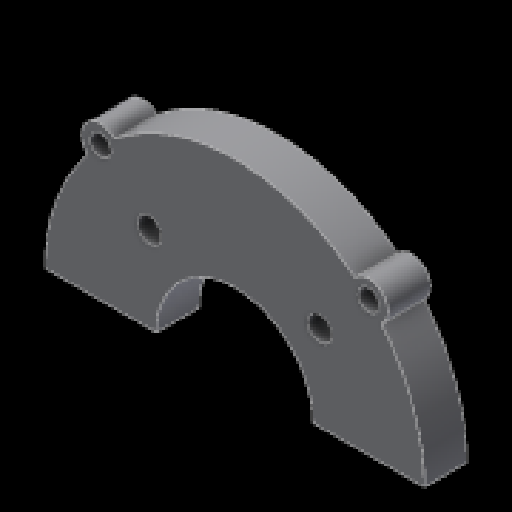
# Autodesk Inventor part: CimCoderMount
Saved by Autodesk Inventor 2025.2 (Build 292293000, 293)
## iProperties
Created: 2026-01-26
Part Number: CimCoderMount
Material: Generic
Document SubType Name: Sheet Metal
Designer: valer
Density: 1 g/cm^3
Appearance: Default
Sheet Metal Rule: Default
Author: valer
Autodesk Inventor part; units mm, degrees
ref_plane "YZ Plane" through (0, 0, 0) normal (1, 0, 0) x (0, 1, 0)
ref_plane "XZ Plane" through (0, 0, 0) normal (0, 1, 0) x (-1, 0, 0)
ref_plane "XY Plane" through (0, 0, 0) normal (0, 0, 1) x (1, 0, 0)
sketch "Base" plane through (0, 0, 0) normal (0, 0, 1) x (1, 0, 0)
  circle A0 centre (0, 0) radius 50.8
  circle A1 centre (0, 0) radius 16.5
  line L0 (-71.12, 0) -> (71.12, 0)
  line L1 (0, -71.12) -> (0, 71.12) construction
  circle A2 centre (-17.9605, 17.9605) radius 2.5527
  circle A3 centre (17.9605, 17.9605) radius 2.5527
  circle A4 centre (17.9605, -17.9605) radius 2.5527
  circle A5 centre (-17.9605, -17.9605) radius 2.5527
  circle A6 centre (0, 0) radius 16 construction
  circle A7 centre (0, 0) radius 40
  line L2 (0, 0) -> (28.2843, 28.2843) construction
  circle A8 centre (28.2843, 28.2843) radius 2.2
  circle A9 centre (-28.2843, 28.2843) radius 2.2
  circle A10 centre (28.2843, -28.2843) radius 2.2
  circle A11 centre (-28.2843, -28.2843) radius 2.2
  circle A12 centre (28.2843, 28.2843) radius 4
  circle A13 centre (17.9605, 17.9605) radius 4
  circle A14 centre (-17.9605, 17.9605) radius 4
  circle A15 centre (-28.2843, 28.2843) radius 4
  line L3 (0, 0) -> (35.921, 35.921)
  line L4 (0, 0) -> (-35.921, 35.921)
  circle A16 centre (28.2843, -28.2843) radius 4
  circle A17 centre (-28.2843, -28.2843) radius 4
  circle A18 centre (17.9605, -17.9605) radius 4
  circle A19 centre (-17.9605, -17.9605) radius 4
  point P0 (-25.4558, 25.4558)
  point P1 (-20.7889, 20.7889)
  point P2 (-15.1321, 15.1321)
  point P3 (-11.6673, 11.6673)
  point P4 (11.6673, 11.6673)
  point P5 (15.1321, 15.1321)
  point P6 (20.7889, 20.7889)
  point P7 (25.4558, 25.4558)
  point P8 (31.1127, 31.1127)
  point P9 (-31.1127, 31.1127)
  point P10 (25.318, 30.9677)
  point P11 (-25.318, 30.9677)
  point P12 (-30.9677, 25.318)
  point P13 (-40, 0)
  point P14 (-16.5, 0)
  point P15 (16.5, 0)
  point P16 (40, 0)
  point P17 (30.9677, 25.318)
  point P18 (30.9677, -25.318)
  point P19 (-30.9677, -25.318)
  point P20 (-25.318, -30.9677)
  point P21 (25.318, -30.9677)
  dimension "d26" = 80
  dimension "d0" = 101.6
  dimension "d25" = 0.5
  dimension "d27" = 4.4
  dimension "d29" = 8
  measures "d0" diameter of A0
  measures "d25" radial gap between concentric circles of A1 A6
  measures "d27" diameter of A8
  measures "d29" diameter of A12
extrude "Plate1" add sketch "Base" along normal blind 9 contours A7 A16 A17 L0 A1 | L0 A1 L3 A13 A12 A7 | L3 A8 A7 A12 | A12 A7 A8 L3 | A7 A15 L4 A14 A1 L0 | A12 L3 A8 A7 | A16 A7 A10 | A7 A10 A16 | L4 A9 A7 A15 | A15 A7 A9 L4 | A12 L3 A13 A1 L4 A14 A15 A7 | A7 A8 L3 A12 | A7 A9 L4 A15 | A17 A7 A11 | A7 A11 A17 | A15 L4 A9 A7 | L3 A3 A13 | A13 L3 A3 | L4 A2 A14 | A14 L4 A2 | A18 | A19
fillet "Fillet2" radius 6 8 edges at (-30.9677, 25.318, 4.5) (-30.9677, -25.318, 4.5) (-25.318, -30.9677, 4.5) (25.318, -30.9677, 4.5) (30.9677, -25.318, 4.5) (30.9677, 25.318, 4.5) (25.318, 30.9677, 4.5) (-25.318, 30.9677, 4.5)
equation "\"d28\" = Thickness"
equation "\"BendRadius\" = Thickness"
equation "\"BendReliefWidth\" = Thickness"
equation "\"BendReliefDepth\" = 0.5 * Thickness"
equation "\"CornerReliefSize\" = 4 * Thickness"
equation "\"MinimumRemnant\" = 2 * Thickness"
equation "\"TransitionRadius\" = BendRadius"
equation "\"JacobiRadiusSize\" = BendRadius"
equation "\"GapSize\" = Thickness"
equation "\"Thickness\" = 9"
body "Solid2"
